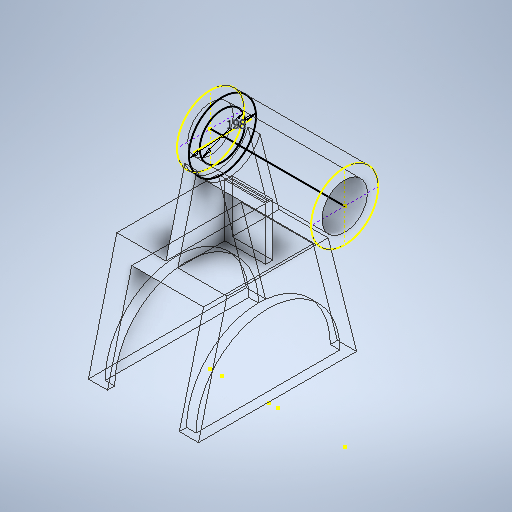
# Autodesk Inventor part: Bai_16
Saved by Autodesk Inventor 2025.1 (Build 291241000, 241)
## iProperties
Created: 2024-10-03
Part Number: Bai_16
Material: Generic
Document SubType Name: Modeling
Designer: msi
Density: 1 g/cm^3
Appearance: Default
Author: msi
Autodesk Inventor part; units mm, degrees
ref_plane "YZ Plane" through (0, 0, 0) normal (1, 0, 0) x (0, 1, 0)
ref_plane "XZ Plane" through (0, 0, 0) normal (0, 1, 0) x (-1, 0, 0)
ref_plane "XY Plane" through (0, 0, 0) normal (0, 0, 1) x (1, 0, 0)
sketch "Sketch1" plane through (0, 0, 0) normal (1, 0, 0) x (0, 1, 0)
  line L0 (0, 33) -> (0, -33)
  line L1 (47.2724, 0) -> (-31.6075, 0)
  line L2 (0, 33) -> (4, 33)
  line L3 (4, 33) -> (4, -33)
  line L4 (4, -33) -> (0, -33)
  line L5 (87, 12) -> (87, -12)
  line L6 (87, 12) -> (4, 33)
  line L7 (87, -12) -> (4, -33)
  line L8 (51, 21.1084) -> (51, -21.1084)
  circle A0 centre (4, 0) radius 24 construction
  circle A1 centre (4, 0) radius 30 construction
  arc A2 (4, -24) -> (4, 24) centre (4, 0) ccw
  arc A3 (4, -30) -> (4, 30) centre (4, 0) ccw
  point P0 (0, 0)
  dimension "d9" = 48
  dimension "d0" = 66
  dimension "d1" = 4
  dimension "d2" = 24
  dimension "d3" = 87
  dimension "d4" = 36
  dimension "d10" = 60
  constraints: 18 end point, 6 point on circle, 6 point on line, 4 horizontal, 4 vertical, 3 centre point, 3 coincident, 2 symmetric about line, 1 midpoint, 1 perpendicular, 1 vertical alignment, 3 other
  measures "d0" distance of L0.start L0.end
  measures "d1" distance of L0.start L2.end
  measures "d2" distance of L5.start L5.end
  measures "d3" distance between parallel lines of L0 L5
  measures "d4" distance between parallel lines of L8 L5
  measures "d10" diameter of A1
extrude "Extrusion1" add sketch "Sketch1" along normal mid plane 46 contours L6 L8 L7 L3 A3 | L3 A2 L1 | L1 A2 L3 | A3 L1 A2 L3 | L1 A3 L3 A2
extrude "Extrusion2" add sketch "Sketch1" along normal mid plane 5 contours L6 L5 L7 L8
sketch "Sketch2" plane through (0, 0, 0) normal (0, 0, 1) x (1, 0, 0)
  line L0 (-2.5, 87) -> (2.5, 87) projected
  line L1 (0, 87) -> (0, 0)
  line L2 (-15, 44) -> (15, 44)
  line L3 (15, 44) -> (15, 4)
  line L4 (15, 4) -> (-15, 4)
  line L5 (-15, 4) -> (-15, 44)
  line L6 (-23, 4) -> (23, 4) projected
  dimension "d13" = 30
  dimension "d14" = 40
  constraints: 10 end point, 2 collinear, 2 parallel, 1 horizontal, 1 midpoint, 1 perpendicular, 1 symmetric about line, 1 vertical
  measures "d13" distance of L2.start L2.end
  measures "d14" distance of L2.end L3.end
extrude "Extrusion4" cut sketch "Sketch2" along normal mid plane 66
sketch "Sketch3" plane through (0, 0, 0) normal (1, 0, 0) x (0, 1, 0)
  line L0 (87, -12) -> (87, 12) projected
  circle A0 centre (87, 0) radius 9.5
  circle A1 centre (87, 0) radius 14
  point P0 (0, 0)
  dimension "d17" = 19
  dimension "d18" = 28
  constraints: 2 centre point, 1 coincident, 1 midpoint
  measures "d17" diameter of A0
  measures "d18" diameter of A1
extrude "Extrusion5" add sketch "Sketch3" along normal blind 51 and the other way blind 5
sketch "Sketch4" plane through (0, 0, 0) normal (1, 0, 0) x (0, 1, 0)
  line L0 (87, 9.5) -> (87, -9.5) projected
  circle A0 centre (87, 0) radius 9.5
  point P0 (0, 0)
  constraints: 1 midpoint, 3 other
extrude "Extrusion6" cut sketch "Sketch4" along normal blind 51 and the other way blind 5 contours L0 A0 picked at (82.8782, 1.7989)
extrude "Extrusion7" cut sketch "Sketch1" along normal mid plane 38 contours L3 A2 L1 | L1 A2 L3 | A3 L1 A2 L3 | L1 A3 L3 A2
sketch "Sketch5" plane through (0, 0, 0) normal (0, 0, 1) x (1, 0, 0)
  line L0 (2.5, 73) -> (19.5, 73)
  line L1 (19.5, 73) -> (19.5, 51)
  line L2 (19.5, 51) -> (2.5, 51)
  line L3 (2.5, 51) -> (2.5, 73)
  line L4 (23, 51) -> (2.5, 51) construction
  line L5 (2.5, 51) -> (0, 51) construction
  line L6 (0, 87.0731) -> (77.1013, 87.0731) construction
  line L7 (0, 87.0731) -> (36, 87.0731)
  point P0 (0, 0)
  dimension "d29" = 22
  dimension "d30" = 17
  dimension "d31" = 36
  constraints: 14 end point, 3 horizontal, 2 parallel, 1 collinear, 1 perpendicular, 1 point on line
  measures "d29" distance of L0.end L1.end
  measures "d30" distance of L2.end L1.end
  measures "d31" distance of L6.start L7.end
extrude "Extrusion8" add sketch "Sketch5" along normal mid plane 3
sketch "Sketch6" plane through (19.5, 51, 1.5) normal (1, 0, 0) x (0, 0, -1)
  point P0 (1.5, -51)
sketch "Sketch7" plane through (-5, 87, 0) normal (-1, 0, 0) x (0, 0, 1)
  point P0 (0, -87)
sketch "Sketch8" plane through (0, 0, 0) normal (0, 0, 1) x (1, 0, 0)
  line L0 (-5, 101) -> (-5, 73) construction
  line L1 (-5, 87) -> (51, 87)
  line L2 (51, 73) -> (51, 101) construction
  point P0 (0, 0)
  constraints: 2 end point, 2 midpoint
sketch "Sketch9" plane through (23, 0, 0) normal (1, 0, 0) x (0, 0, -1)
  point P0 (0, 0)
sketch "Sketch10" plane through (51, 87, 0) normal (1, 0, 0) x (0, 0, -1)
  circle A0 centre (0, 0) radius 14 projected
  line L0 (-14, 0) -> (14, 0) construction
  point P0 (0, -87)
  constraints: 2 end point, 2 point on circle, 1 horizontal
sketch "Sketch11" plane through (-5, 87, 0) normal (-1, 0, 0) x (0, 0, 1)
  circle A0 centre (0, 0) radius 14 projected
  line L0 (-14, 0) -> (14, 0) construction
  point P0 (0, -87)
  constraints: 2 end point, 2 point on circle, 1 horizontal
body "Solid1"
